Autodesk Fusion 360 part; units mm, degrees
(part 3 of 5)
  spline S134 degree 5 poles (-1.9006, 45.6475) (-1.9013, 45.6491) (-1.9092, 45.6653) (-1.9241, 45.6961) (-1.9463, 45.7414) (-1.9758, 45.8013) (-2.0121, 45.8741) (-2.0487, 45.9468) (-2.0857, 46.0195) (-2.123, 46.092) (-2.1607, 46.1645) (-2.1987, 46.2369) (-2.2371, 46.3092) (-2.2758, 46.3814) (-2.3148, 46.4536) (-2.3542, 46.5256) (-2.3938, 46.5976) (-2.4339, 46.6694) (-2.4742, 46.7412) (-2.5149, 46.8129) (-2.5559, 46.8845) (-2.5972, 46.956) (-2.6305, 47.0132) (-2.6556, 47.056) (-2.6724, 47.0845) (-2.6809, 47.0988) knots 0.712736 0.712736 0.712736 0.712736 0.712736 0.712736 0.714286 0.728571 0.742857 0.757143 0.771429 0.785714 0.8 0.814286 0.828571 0.842857 0.857143 0.871429 0.885714 0.9 0.914286 0.928571 0.942857 0.957143 0.971429 0.985714 1 1 1 1 1 1
  arc A101 (-2.6809, 47.0988) -> (-3.2433, 47.0634) centre (0, 0) ccw
  spline S135 degree 5 poles (-44.9524, 14.3096) (-44.9406, 14.2979) (-44.9172, 14.2745) (-44.882, 14.2396) (-44.8349, 14.1931) (-44.7759, 14.1353) (-44.7168, 14.0778) (-44.6574, 14.0206) (-44.5979, 13.9636) (-44.5383, 13.907) (-44.4785, 13.8506) (-44.4185, 13.7946) (-44.3583, 13.7389) (-44.298, 13.6834) (-44.2375, 13.6283) (-44.1768, 13.5735) (-44.116, 13.5189) (-44.055, 13.4647) (-43.9938, 13.4109) (-43.9325, 13.3573) (-43.871, 13.3041) (-43.8203, 13.2606) (-43.7819, 13.2278) (-43.7558, 13.2057) (-43.7421, 13.1941) (-43.7407, 13.1929) knots -1 -1 -1 -1 -1 -1 -0.985714 -0.971429 -0.957143 -0.942857 -0.928571 -0.914286 -0.9 -0.885714 -0.871429 -0.857143 -0.842857 -0.828571 -0.814286 -0.8 -0.785714 -0.771429 -0.757143 -0.742857 -0.728571 -0.714286 -0.712736 -0.712736 -0.712736 -0.712736 -0.712736 -0.712736
  spline S136 degree 5 poles (-22.8544, -39.5598) (-22.8546, -39.5616) (-22.8567, -39.5795) (-22.8606, -39.6135) (-22.8662, -39.6636) (-22.8733, -39.73) (-22.8817, -39.8109) (-22.8898, -39.892) (-22.8975, -39.9731) (-22.9048, -40.0544) (-22.9118, -40.1357) (-22.9185, -40.2172) (-22.9249, -40.2988) (-22.9309, -40.3805) (-22.9366, -40.4624) (-22.942, -40.5443) (-22.947, -40.6263) (-22.9517, -40.7084) (-22.9561, -40.7907) (-22.9602, -40.873) (-22.964, -40.9554) (-22.9674, -41.0379) (-22.9699, -41.104) (-22.9716, -41.1536) (-22.9727, -41.1867) (-22.9733, -41.2033) knots 0.712736 0.712736 0.712736 0.712736 0.712736 0.712736 0.714286 0.728571 0.742857 0.757143 0.771429 0.785714 0.8 0.814286 0.828571 0.842857 0.857143 0.871429 0.885714 0.9 0.914286 0.928571 0.942857 0.957143 0.971429 0.985714 1 1 1 1 1 1
  spline S137 degree 5 poles (22.4794, 41.4748) (22.4657, 41.4655) (22.4383, 41.4468) (22.3974, 41.4188) (22.3429, 41.3812) (22.2751, 41.3341) (22.2075, 41.2868) (22.1402, 41.2392) (22.0731, 41.1915) (22.0063, 41.1435) (21.9397, 41.0953) (21.8734, 41.0468) (21.8074, 40.9982) (21.7417, 40.9493) (21.6762, 40.9002) (21.6109, 40.8509) (21.546, 40.8014) (21.4813, 40.7516) (21.4169, 40.7016) (21.3528, 40.6514) (21.289, 40.601) (21.2368, 40.5594) (21.1974, 40.5278) (21.1708, 40.5063) (21.1568, 40.495) (21.1555, 40.4939) knots -1 -1 -1 -1 -1 -1 -0.985714 -0.971429 -0.957143 -0.942857 -0.928571 -0.914286 -0.9 -0.885714 -0.871429 -0.857143 -0.842857 -0.828571 -0.814286 -0.8 -0.785714 -0.771429 -0.757143 -0.742857 -0.728571 -0.714286 -0.712736 -0.712736 -0.712736 -0.712736 -0.712736 -0.712736
  spline S138 degree 5 poles (-17.628, 43.7577) (-17.6295, 43.7412) (-17.6326, 43.7082) (-17.6371, 43.6588) (-17.6429, 43.5929) (-17.6498, 43.5106) (-17.6564, 43.4284) (-17.6627, 43.3462) (-17.6686, 43.264) (-17.6743, 43.182) (-17.6795, 43.1) (-17.6845, 43.018) (-17.6891, 42.9361) (-17.6933, 42.8543) (-17.6973, 42.7726) (-17.7008, 42.6909) (-17.7041, 42.6093) (-17.707, 42.5277) (-17.7095, 42.4462) (-17.7117, 42.3648) (-17.7135, 42.2835) (-17.7147, 42.2168) (-17.7154, 42.1663) (-17.7158, 42.1321) (-17.716, 42.1141) (-17.7161, 42.1123) knots -1 -1 -1 -1 -1 -1 -0.985714 -0.971429 -0.957143 -0.942857 -0.928571 -0.914286 -0.9 -0.885714 -0.871429 -0.857143 -0.842857 -0.828571 -0.814286 -0.8 -0.785714 -0.771429 -0.757143 -0.742857 -0.728571 -0.714286 -0.712736 -0.712736 -0.712736 -0.712736 -0.712736 -0.712736
  spline S139 degree 3 poles (-42.1123, 17.7161) (-42.0459, 17.7168) (-41.9803, 17.7305) (-41.858, 17.7822) (-41.8024, 17.8198) (-41.7089, 17.9141) (-41.6718, 17.97) (-41.6211, 18.0927) (-41.608, 18.1585) (-41.6077, 18.2913) (-41.6206, 18.3571) (-41.6685, 18.4748) (-41.7013, 18.5264) (-41.7423, 18.5711) knots 0 0 0 0 0.019923 0.019923 0.039846 0.039846 0.059769 0.059769 0.079691 0.079691 0.099614 0.099614 0.117812 0.117812 0.117812 0.117812
  arc A102 (-8.5628, 46.3914) -> (-9.1163, 46.2858) centre (0, 0) ccw
  spline S140 degree 3 poles (27.6324, 36.3835) (27.6166, 36.319) (27.6135, 36.252) (27.6332, 36.1207) (27.6558, 36.0575) (27.7239, 35.9435) (27.7688, 35.8937) (27.8751, 35.8141) (27.9355, 35.785) (28.0641, 35.7517) (28.131, 35.7477) (28.2569, 35.7649) (28.3151, 35.7838) (28.3685, 35.8125) knots 0 0 0 0 0.019923 0.019923 0.039846 0.039846 0.059769 0.059769 0.079691 0.079691 0.099614 0.099614 0.117812 0.117812 0.117812 0.117812
  spline S141 degree 5 poles (-45.5258, 3.8356) (-45.5274, 3.835) (-45.5445, 3.8292) (-45.5769, 3.8183) (-45.6247, 3.802) (-45.6878, 3.7802) (-45.7646, 3.7533) (-45.8413, 3.7261) (-45.918, 3.6985) (-45.9947, 3.6706) (-46.0713, 3.6423) (-46.1479, 3.6137) (-46.2244, 3.5847) (-46.3009, 3.5553) (-46.3774, 3.5256) (-46.4538, 3.4956) (-46.5301, 3.4653) (-46.6065, 3.4346) (-46.6827, 3.4035) (-46.759, 3.3722) (-46.8351, 3.3405) (-46.9113, 3.3084) (-46.9721, 3.2825) (-47.0178, 3.263) (-47.0482, 3.2499) (-47.0634, 3.2433) knots 0.712736 0.712736 0.712736 0.712736 0.712736 0.712736 0.714286 0.728571 0.742857 0.757143 0.771429 0.785714 0.8 0.814286 0.828571 0.842857 0.857143 0.871429 0.885714 0.9 0.914286 0.928571 0.942857 0.957143 0.971429 0.985714 1 1 1 1 1 1
  spline S142 degree 5 poles (-42.1123, 17.7161) (-42.1141, 17.716) (-42.1321, 17.7158) (-42.1663, 17.7154) (-42.2168, 17.7147) (-42.2835, 17.7135) (-42.3648, 17.7117) (-42.4462, 17.7095) (-42.5277, 17.707) (-42.6093, 17.7041) (-42.6909, 17.7008) (-42.7726, 17.6973) (-42.8543, 17.6933) (-42.9361, 17.6891) (-43.018, 17.6845) (-43.1, 17.6795) (-43.182, 17.6743) (-43.264, 17.6686) (-43.3462, 17.6627) (-43.4284, 17.6564) (-43.5106, 17.6498) (-43.5929, 17.6429) (-43.6588, 17.6371) (-43.7082, 17.6326) (-43.7412, 17.6295) (-43.7577, 17.628) knots 0.712736 0.712736 0.712736 0.712736 0.712736 0.712736 0.714286 0.728571 0.742857 0.757143 0.771429 0.785714 0.8 0.814286 0.828571 0.842857 0.857143 0.871429 0.885714 0.9 0.914286 0.928571 0.942857 0.957143 0.971429 0.985714 1 1 1 1 1 1
  spline S143 degree 3 poles (22.8544, 39.5598) (22.8468, 39.4939) (22.8522, 39.427) (22.8882, 39.2992) (22.9185, 39.2394) (23.0004, 39.1348) (23.0511, 39.091) (23.1666, 39.0253) (23.2302, 39.0041) (23.3619, 38.9871) (23.4288, 38.9916) (23.5515, 39.0245) (23.6069, 39.0505) (23.6563, 39.0856) knots 0 0 0 0 0.019923 0.019923 0.039846 0.039846 0.059769 0.059769 0.079691 0.079691 0.099614 0.099614 0.117812 0.117812 0.117812 0.117812
  spline S144 degree 5 poles (22.8544, 39.5598) (22.8546, 39.5616) (22.8567, 39.5795) (22.8606, 39.6135) (22.8662, 39.6636) (22.8733, 39.73) (22.8817, 39.8109) (22.8898, 39.892) (22.8975, 39.9731) (22.9048, 40.0544) (22.9118, 40.1357) (22.9185, 40.2172) (22.9249, 40.2988) (22.9309, 40.3805) (22.9366, 40.4624) (22.942, 40.5443) (22.947, 40.6263) (22.9517, 40.7084) (22.9561, 40.7907) (22.9602, 40.873) (22.964, 40.9554) (22.9674, 41.0379) (22.9699, 41.104) (22.9716, 41.1536) (22.9727, 41.1867) (22.9733, 41.2033) knots 0.712736 0.712736 0.712736 0.712736 0.712736 0.712736 0.714286 0.728571 0.742857 0.757143 0.771429 0.785714 0.8 0.814286 0.828571 0.842857 0.857143 0.871429 0.885714 0.9 0.914286 0.928571 0.942857 0.957143 0.971429 0.985714 1 1 1 1 1 1
  spline S145 degree 3 poles (-22.8544, -39.5598) (-22.8468, -39.4939) (-22.8522, -39.427) (-22.8882, -39.2992) (-22.9185, -39.2394) (-23.0004, -39.1348) (-23.0511, -39.091) (-23.1666, -39.0253) (-23.2302, -39.0041) (-23.3619, -38.9871) (-23.4288, -38.9916) (-23.5515, -39.0245) (-23.6069, -39.0505) (-23.6563, -39.0856) knots 0 0 0 0 0.019923 0.019923 0.039846 0.039846 0.059769 0.059769 0.079691 0.079691 0.099614 0.099614 0.117812 0.117812 0.117812 0.117812
  spline S146 degree 5 poles (-44.0007, 12.2983) (-44.0024, 12.2981) (-44.0202, 12.2956) (-44.0541, 12.2909) (-44.1041, 12.2838) (-44.1702, 12.2743) (-44.2506, 12.2623) (-44.3311, 12.2499) (-44.4116, 12.2372) (-44.4922, 12.2241) (-44.5727, 12.2107) (-44.6533, 12.1969) (-44.734, 12.1828) (-44.8146, 12.1683) (-44.8953, 12.1534) (-44.9759, 12.1383) (-45.0566, 12.1228) (-45.1374, 12.1069) (-45.2181, 12.0907) (-45.2989, 12.0742) (-45.3796, 12.0573) (-45.4604, 12.0401) (-45.525, 12.0261) (-45.5735, 12.0154) (-45.6059, 12.0083) (-45.622, 12.0047) knots 0.712736 0.712736 0.712736 0.712736 0.712736 0.712736 0.714286 0.728571 0.742857 0.757143 0.771429 0.785714 0.8 0.814286 0.828571 0.842857 0.857143 0.871429 0.885714 0.9 0.914286 0.928571 0.942857 0.957143 0.971429 0.985714 1 1 1 1 1 1
  spline S147 degree 5 poles (-6.192, 46.7669) (-6.1976, 46.7513) (-6.2088, 46.7201) (-6.2255, 46.6733) (-6.2475, 46.611) (-6.2747, 46.533) (-6.3015, 46.455) (-6.328, 46.3769) (-6.3542, 46.2988) (-6.3801, 46.2207) (-6.4056, 46.1426) (-6.4307, 46.0645) (-6.4556, 45.9863) (-6.48, 45.9081) (-6.5042, 45.8299) (-6.5279, 45.7517) (-6.5514, 45.6734) (-6.5744, 45.5952) (-6.5972, 45.5169) (-6.6195, 45.4386) (-6.6415, 45.3603) (-6.6593, 45.2959) (-6.6725, 45.2472) (-6.6815, 45.2142) (-6.6861, 45.1968) (-6.6866, 45.1951) knots -1 -1 -1 -1 -1 -1 -0.985714 -0.971429 -0.957143 -0.942857 -0.928571 -0.914286 -0.9 -0.885714 -0.871429 -0.857143 -0.842857 -0.828571 -0.814286 -0.8 -0.785714 -0.771429 -0.757143 -0.742857 -0.728571 -0.714286 -0.712736 -0.712736 -0.712736 -0.712736 -0.712736 -0.712736
  arc A103 (-34.5814, -32.0875) -> (-34.1956, -32.4983) centre (0, 0) ccw
  arc A104 (-27.9562, -37.9991) -> (-27.5003, -38.3303) centre (0, 0) ccw
  spline S148 degree 5 poles (27.5003, 38.3303) (27.4856, 38.3228) (27.4561, 38.3077) (27.4119, 38.285) (27.3532, 38.2546) (27.28, 38.2164) (27.207, 38.1779) (27.1342, 38.1392) (27.0617, 38.1002) (26.9894, 38.0609) (26.9173, 38.0214) (26.8455, 37.9817) (26.7739, 37.9417) (26.7025, 37.9015) (26.6314, 37.861) (26.5605, 37.8202) (26.4899, 37.7792) (26.4195, 37.738) (26.3493, 37.6964) (26.2794, 37.6547) (26.2098, 37.6126) (26.1528, 37.5779) (26.1098, 37.5514) (26.0807, 37.5335) (26.0654, 37.524) (26.0639, 37.5231) knots -1 -1 -1 -1 -1 -1 -0.985714 -0.971429 -0.957143 -0.942857 -0.928571 -0.914286 -0.9 -0.885714 -0.871429 -0.857143 -0.842857 -0.828571 -0.814286 -0.8 -0.785714 -0.771429 -0.757143 -0.742857 -0.728571 -0.714286 -0.712736 -0.712736 -0.712736 -0.712736 -0.712736 -0.712736
  spline S149 degree 5 poles (-3.2433, 47.0634) (-3.2499, 47.0482) (-3.263, 47.0178) (-3.2825, 46.9721) (-3.3084, 46.9113) (-3.3405, 46.8351) (-3.3722, 46.759) (-3.4035, 46.6827) (-3.4346, 46.6065) (-3.4653, 46.5301) (-3.4956, 46.4538) (-3.5256, 46.3774) (-3.5553, 46.3009) (-3.5847, 46.2244) (-3.6137, 46.1479) (-3.6423, 46.0713) (-3.6706, 45.9947) (-3.6985, 45.918) (-3.7261, 45.8413) (-3.7533, 45.7646) (-3.7802, 45.6878) (-3.802, 45.6247) (-3.8183, 45.5769) (-3.8292, 45.5445) (-3.835, 45.5274) (-3.8356, 45.5258) knots -1 -1 -1 -1 -1 -1 -0.985714 -0.971429 -0.957143 -0.942857 -0.928571 -0.914286 -0.9 -0.885714 -0.871429 -0.857143 -0.842857 -0.828571 -0.814286 -0.8 -0.785714 -0.771429 -0.757143 -0.742857 -0.728571 -0.714286 -0.712736 -0.712736 -0.712736 -0.712736 -0.712736 -0.712736
  arc A105 (45.7622, 11.4588) -> (45.622, 12.0047) centre (0, 0) ccw
  spline S150 degree 3 poles (43.7407, 13.1929) (43.69, 13.1501) (43.6482, 13.0977) (43.5869, 12.9798) (43.5681, 12.9155) (43.5562, 12.7832) (43.5632, 12.7165) (43.6024, 12.5896) (43.6342, 12.5306) (43.7186, 12.4281) (43.7704, 12.3855) (43.8824, 12.3255) (43.9406, 12.3066) (44.0007, 12.2983) knots 0 0 0 0 0.019923 0.019923 0.039846 0.039846 0.059769 0.059769 0.079691 0.079691 0.099614 0.099614 0.117812 0.117812 0.117812 0.117812
  spline S151 degree 5 poles (44.7782, 14.8456) (44.7619, 14.8482) (44.7291, 14.8533) (44.6801, 14.8609) (44.6147, 14.8709) (44.533, 14.8829) (44.4513, 14.8947) (44.3697, 14.9061) (44.2881, 14.9172) (44.2065, 14.928) (44.125, 14.9384) (44.0436, 14.9485) (43.9621, 14.9582) (43.8807, 14.9676) (43.7994, 14.9766) (43.7181, 14.9853) (43.6368, 14.9937) (43.5556, 15.0017) (43.4745, 15.0093) (43.3934, 15.0166) (43.3123, 15.0235) (43.2458, 15.0289) (43.1954, 15.0328) (43.1613, 15.0354) (43.1434, 15.0367) (43.1416, 15.0368) knots -1 -1 -1 -1 -1 -1 -0.985714 -0.971429 -0.957143 -0.942857 -0.928571 -0.914286 -0.9 -0.885714 -0.871429 -0.857143 -0.842857 -0.828571 -0.814286 -0.8 -0.785714 -0.771429 -0.757143 -0.742857 -0.728571 -0.714286 -0.712736 -0.712736 -0.712736 -0.712736 -0.712736 -0.712736
  arc A106 (42.8044, 19.8308) -> (42.5645, 20.3407) centre (0, 0) ccw
  line L56 (29.0727, 9.9241) -> (36.6833, 12.3969)
  spline S152 degree 5 poles (44.4828, 10.4204) (44.4842, 10.4215) (44.4987, 10.4322) (44.5261, 10.4526) (44.5665, 10.4829) (44.6198, 10.5231) (44.6845, 10.5724) (44.7491, 10.622) (44.8135, 10.6719) (44.8778, 10.7222) (44.9419, 10.7728) (45.0059, 10.8237) (45.0698, 10.8749) (45.1334, 10.9265) (45.197, 10.9783) (45.2604, 11.0305) (45.3236, 11.083) (45.3867, 11.1357) (45.4497, 11.1888) (45.5125, 11.2422) (45.5751, 11.2959) (45.6376, 11.3499) (45.6875, 11.3933) (45.7249, 11.426) (45.7497, 11.4479) (45.7622, 11.4588) knots 0.712736 0.712736 0.712736 0.712736 0.712736 0.712736 0.714286 0.728571 0.742857 0.757143 0.771429 0.785714 0.8 0.814286 0.828571 0.842857 0.857143 0.871429 0.885714 0.9 0.914286 0.928571 0.942857 0.957143 0.971429 0.985714 1 1 1 1 1 1
  line L57 (23.3964, 19.6289) -> (29.5622, 24.7297)
  line L58 (25.6911, 16.6409) -> (32.4476, 20.9287)
  spline S153 degree 5 poles (40.4939, 21.1555) (40.495, 21.1568) (40.5063, 21.1708) (40.5278, 21.1974) (40.5594, 21.2368) (40.601, 21.289) (40.6514, 21.3528) (40.7016, 21.4169) (40.7516, 21.4813) (40.8014, 21.546) (40.8509, 21.6109) (40.9002, 21.6762) (40.9493, 21.7417) (40.9982, 21.8074) (41.0468, 21.8734) (41.0953, 21.9397) (41.1435, 22.0063) (41.1915, 22.0731) (41.2392, 22.1402) (41.2868, 22.2075) (41.3341, 22.2751) (41.3812, 22.3429) (41.4188, 22.3974) (41.4468, 22.4383) (41.4655, 22.4657) (41.4748, 22.4794) knots 0.712736 0.712736 0.712736 0.712736 0.712736 0.712736 0.714286 0.728571 0.742857 0.757143 0.771429 0.785714 0.8 0.814286 0.828571 0.842857 0.857143 0.871429 0.885714 0.9 0.914286 0.928571 0.942857 0.957143 0.971429 0.985714 1 1 1 1 1 1
  arc A107 (-11.213, -27.5925) -> (-9.5008, -28.2786) centre (0.7975, -0.1016) ccw
  spline S154 degree 3 poles (39.0856, 23.6563) (39.0471, 23.6022) (39.0196, 23.541) (38.9896, 23.4117) (38.9874, 23.3447) (39.0087, 23.2136) (39.0321, 23.1507) (39.1016, 23.0376) (39.1471, 22.9883) (39.2544, 22.91) (39.3152, 22.8817) (39.4386, 22.8514) (39.4996, 22.8475) (39.5598, 22.8544) knots 0 0 0 0 0.019923 0.019923 0.039846 0.039846 0.059769 0.059769 0.079691 0.079691 0.099614 0.099614 0.117812 0.117812 0.117812 0.117812
  arc A108 (43.9652, 17.104) -> (43.7577, 17.628) centre (0, 0) ccw
  spline S155 degree 3 poles (42.826, 15.9134) (42.7781, 15.8674) (42.7397, 15.8125) (42.6859, 15.6911) (42.6712, 15.6257) (42.6676, 15.4929) (42.6788, 15.4268) (42.7258, 15.3026) (42.7613, 15.2457) (42.852, 15.1487) (42.9064, 15.1095) (43.0219, 15.0565) (43.0811, 15.0413) (43.1416, 15.0368) knots 0 0 0 0 0.019923 0.019923 0.039846 0.039846 0.059769 0.059769 0.079691 0.079691 0.099614 0.099614 0.117812 0.117812 0.117812 0.117812
  arc A109 (33.573, 19.1277) -> (32.4476, 20.9287) centre (0.7975, -0.1016) ccw
  spline S156 degree 5 poles (45.6768, -0.9694) (45.6784, -0.9687) (45.695, -0.9619) (45.7267, -0.9489) (45.7734, -0.9297) (45.835, -0.904) (45.9099, -0.8723) (45.9848, -0.8404) (46.0596, -0.808) (46.1344, -0.7753) (46.2091, -0.7423) (46.2837, -0.7089) (46.3583, -0.6751) (46.4328, -0.641) (46.5072, -0.6066) (46.5816, -0.5719) (46.6559, -0.5368) (46.7302, -0.5013) (46.8043, -0.4656) (46.8784, -0.4295) (46.9525, -0.3931) (47.0264, -0.3563) (47.0856, -0.3267) (47.1299, -0.3043) (47.1594, -0.2893) (47.1742, -0.2818) knots 0.712736 0.712736 0.712736 0.712736 0.712736 0.712736 0.714286 0.728571 0.742857 0.757143 0.771429 0.785714 0.8 0.814286 0.828571 0.842857 0.857143 0.871429 0.885714 0.9 0.914286 0.928571 0.942857 0.957143 0.971429 0.985714 1 1 1 1 1 1
  line L59 (27.5932, 13.3889) -> (34.8338, 16.7961)
  line L60 (28.3716, 11.7167) -> (35.7247, 14.8682)
  arc A110 (-47.1742, 0.2818) -> (-47.1742, -0.2818) centre (0, 0) ccw
  arc A111 (37.3255, 10.3726) -> (36.6833, 12.3969) centre (0.7975, -0.1016) ccw
  spline S157 degree 5 poles (42.826, 15.9134) (42.8273, 15.9146) (42.8403, 15.9271) (42.8649, 15.9508) (42.9012, 15.9859) (42.9491, 16.0325) (43.0071, 16.0895) (43.065, 16.1468) (43.1226, 16.2044) (43.1801, 16.2623) (43.2374, 16.3206) (43.2945, 16.3791) (43.3514, 16.4379) (43.4081, 16.497) (43.4646, 16.5564) (43.521, 16.6161) (43.5772, 16.6761) (43.6332, 16.7364) (43.689, 16.7969) (43.7446, 16.8578) (43.8, 16.9189) (43.8553, 16.9803) (43.8993, 17.0296) (43.9323, 17.0668) (43.9542, 17.0916) (43.9652, 17.104) knots 0.712736 0.712736 0.712736 0.712736 0.712736 0.712736 0.714286 0.728571 0.742857 0.757143 0.771429 0.785714 0.8 0.814286 0.828571 0.842857 0.857143 0.871429 0.885714 0.9 0.914286 0.928571 0.942857 0.957143 0.971429 0.985714 1 1 1 1 1 1
  line L61 (0.7975, -0.1016) -> (38, -0.1016) construction
  line L62 (24.5662, 18.2028) -> (30.9045, 23.0839)
  arc A112 (44.9524, 14.3096) -> (44.7782, 14.8456) centre (0, 0) ccw
  spline S158 degree 5 poles (41.7423, 18.5711) (41.7435, 18.5724) (41.7557, 18.5856) (41.7788, 18.6109) (41.8128, 18.6481) (41.8576, 18.6976) (41.912, 18.7582) (41.9661, 18.819) (42.02, 18.8801) (42.0738, 18.9415) (42.1273, 19.0032) (42.1806, 19.0652) (42.2337, 19.1275) (42.2866, 19.1901) (42.3393, 19.2529) (42.3918, 19.3161) (42.4441, 19.3794) (42.4962, 19.4431) (42.5481, 19.5071) (42.5997, 19.5713) (42.6512, 19.6357) (42.7025, 19.7005) (42.7434, 19.7525) (42.7739, 19.7916) (42.7943, 19.8177) (42.8044, 19.8308) knots 0.712736 0.712736 0.712736 0.712736 0.712736 0.712736 0.714286 0.728571 0.742857 0.757143 0.771429 0.785714 0.8 0.814286 0.828571 0.842857 0.857143 0.871429 0.885714 0.9 0.914286 0.928571 0.942857 0.957143 0.971429 0.985714 1 1 1 1 1 1
  line L63 (26.6729, 15.0794) -> (33.573, 19.1277)
  spline S159 degree 5 poles (45.4381, 4.7631) (45.4396, 4.7639) (45.4553, 4.7728) (45.4851, 4.7896) (45.5289, 4.8146) (45.5869, 4.8478) (45.6572, 4.8886) (45.7275, 4.9297) (45.7977, 4.9712) (45.8678, 5.013) (45.9377, 5.0551) (46.0076, 5.0976) (46.0774, 5.1404) (46.147, 5.1836) (46.2165, 5.2271) (46.286, 5.2709) (46.3553, 5.315) (46.4245, 5.3595) (46.4936, 5.4042) (46.5626, 5.4493) (46.6315, 5.4947) (46.7003, 5.5405) (46.7552, 5.5773) (46.7964, 5.6051) (46.8238, 5.6236) (46.8375, 5.6329) knots 0.712736 0.712736 0.712736 0.712736 0.712736 0.712736 0.714286 0.728571 0.742857 0.757143 0.771429 0.785714 0.8 0.814286 0.828571 0.842857 0.857143 0.871429 0.885714 0.9 0.914286 0.928571 0.942857 0.957143 0.971429 0.985714 1 1 1 1 1 1
  arc A113 (47.1742, -0.2818) -> (47.1742, 0.2818) centre (0, 0) ccw
  arc A114 (38.3502, 5.7119) -> (37.9668, 7.8007) centre (0.7975, -0.1016) ccw
  spline S160 degree 5 poles (47.0634, 3.2433) (47.0482, 3.2499) (47.0178, 3.263) (46.9721, 3.2825) (46.9113, 3.3084) (46.8351, 3.3405) (46.759, 3.3722) (46.6827, 3.4035) (46.6065, 3.4346) (46.5301, 3.4653) (46.4538, 3.4956) (46.3774, 3.5256) (46.3009, 3.5553) (46.2244, 3.5847) (46.1479, 3.6137) (46.0713, 3.6423) (45.9947, 3.6706) (45.918, 3.6985) (45.8413, 3.7261) (45.7646, 3.7533) (45.6878, 3.7802) (45.6247, 3.802) (45.5769, 3.8183) (45.5445, 3.8292) (45.5274, 3.835) (45.5258, 3.8356) knots -1 -1 -1 -1 -1 -1 -0.985714 -0.971429 -0.957143 -0.942857 -0.928571 -0.914286 -0.9 -0.885714 -0.871429 -0.857143 -0.842857 -0.828571 -0.814286 -0.8 -0.785714 -0.771429 -0.757143 -0.742857 -0.728571 -0.714286 -0.712736 -0.712736 -0.712736 -0.712736 -0.712736 -0.712736
  arc A115 (30.4444, 4.488) -> (30.1063, 6.3012) centre (0.7975, -0.1016) ccw
  spline S161 degree 3 poles (45.4381, 4.7631) (45.3802, 4.7304) (45.3293, 4.6868) (45.2471, 4.5825) (45.2165, 4.5229) (45.18, 4.3952) (45.1744, 4.3283) (45.1891, 4.1963) (45.2093, 4.1324) (45.273, 4.0159) (45.316, 3.9644) (45.4147, 3.8844) (45.4683, 3.8549) (45.5258, 3.8356) knots 0 0 0 0 0.019923 0.019923 0.039846 0.039846 0.059769 0.059769 0.079691 0.079691 0.099614 0.099614 0.117812 0.117812 0.117812 0.117812
  arc A116 (47.0988, 2.6809) -> (47.0634, 3.2433) centre (0, 0) ccw
  spline S162 degree 5 poles (45.0493, 7.6067) (45.0508, 7.6077) (45.0659, 7.6175) (45.0946, 7.6362) (45.1368, 7.6639) (45.1925, 7.7007) (45.2602, 7.7458) (45.3278, 7.7912) (45.3952, 7.837) (45.4625, 7.8831) (45.5297, 7.9296) (45.5967, 7.9764) (45.6637, 8.0235) (45.7305, 8.0709) (45.7971, 8.1187) (45.8637, 8.1668) (45.9301, 8.2152) (45.9964, 8.2639) (46.0625, 8.3129) (46.1286, 8.3623) (46.1945, 8.4119) (46.2602, 8.4619) (46.3128, 8.5021) (46.3521, 8.5324) (46.3783, 8.5526) (46.3914, 8.5628) knots 0.712736 0.712736 0.712736 0.712736 0.712736 0.712736 0.714286 0.728571 0.742857 0.757143 0.771429 0.785714 0.8 0.814286 0.828571 0.842857 0.857143 0.871429 0.885714 0.9 0.914286 0.928571 0.942857 0.957143 0.971429 0.985714 1 1 1 1 1 1
  spline S163 degree 5 poles (46.2858, 9.1163) (46.2699, 9.121) (46.2381, 9.1301) (46.1903, 9.1438) (46.1267, 9.1619) (46.0472, 9.1841) (45.9676, 9.206) (45.8881, 9.2276) (45.8085, 9.2488) (45.7289, 9.2697) (45.6494, 9.2903) (45.5698, 9.3105) (45.4902, 9.3303) (45.4106, 9.3498) (45.3311, 9.369) (45.2515, 9.3878) (45.1719, 9.4063) (45.0924, 9.4244) (45.0128, 9.4422) (44.9333, 9.4596) (44.8537, 9.4766) (44.7884, 9.4903) (44.7389, 9.5005) (44.7054, 9.5073) (44.6878, 9.5109) (44.686, 9.5112) knots -1 -1 -1 -1 -1 -1 -0.985714 -0.971429 -0.957143 -0.942857 -0.928571 -0.914286 -0.9 -0.885714 -0.871429 -0.857143 -0.842857 -0.828571 -0.814286 -0.8 -0.785714 -0.771429 -0.757143 -0.742857 -0.728571 -0.714286 -0.712736 -0.712736 -0.712736 -0.712736 -0.712736 -0.712736
  spline S164 degree 5 poles (47.1742, 0.2818) (47.1594, 0.2893) (47.1299, 0.3043) (47.0856, 0.3267) (47.0264, 0.3563) (46.9525, 0.3931) (46.8784, 0.4295) (46.8043, 0.4656) (46.7302, 0.5013) (46.6559, 0.5368) (46.5816, 0.5719) (46.5072, 0.6066) (46.4328, 0.641) (46.3583, 0.6751) (46.2837, 0.7089) (46.2091, 0.7423) (46.1344, 0.7753) (46.0596, 0.808) (45.9848, 0.8404) (45.9099, 0.8723) (45.835, 0.904) (45.7734, 0.9297) (45.7267, 0.9489) (45.695, 0.9619) (45.6784, 0.9687) (45.6768, 0.9694) knots -1 -1 -1 -1 -1 -1 -0.985714 -0.971429 -0.957143 -0.942857 -0.928571 -0.914286 -0.9 -0.885714 -0.871429 -0.857143 -0.842857 -0.828571 -0.814286 -0.8 -0.785714 -0.771429 -0.757143 -0.742857 -0.728571 -0.714286 -0.712736 -0.712736 -0.712736 -0.712736 -0.712736 -0.712736
  spline S165 degree 3 poles (44.4828, 10.4204) (44.4295, 10.3808) (44.3845, 10.3311) (44.3159, 10.2174) (44.2931, 10.1543) (44.2729, 10.0231) (44.2757, 9.9561) (44.3069, 9.827) (44.3349, 9.7661) (44.4127, 9.6584) (44.4618, 9.6127) (44.5698, 9.5457) (44.6266, 9.5232) (44.686, 9.5112) knots 0 0 0 0 0.019923 0.019923 0.039846 0.039846 0.059769 0.059769 0.079691 0.079691 0.099614 0.099614 0.117812 0.117812 0.117812 0.117812
  line L64 (30.6777, 2.5774) -> (38.6641, 3.0798)
  line L65 (30.1063, 6.3012) -> (37.9668, 7.8007)
  line L66 (30.4444, 4.488) -> (38.3502, 5.7119)
  line L67 (30.7858, 0.736) -> (38.7827, 0.9594)
  arc A117 (38.7827, 0.9594) -> (38.6641, 3.0798) centre (0.7975, -0.1016) ccw
  arc A118 (46.3914, 8.5628) -> (46.2858, 9.1163) centre (0, 0) ccw
  arc A119 (29.6354, 8.1675) -> (29.0727, 9.9241) centre (0.7975, -0.1016) ccw
  spline S166 degree 3 poles (45.0493, 7.6067) (44.9937, 7.5705) (44.9456, 7.5238) (44.87, 7.4146) (44.8433, 7.3531) (44.8149, 7.2234) (44.8135, 7.1563) (44.8365, 7.0255) (44.8606, 6.963) (44.9315, 6.8507) (44.9776, 6.802) (45.0812, 6.7283) (45.1365, 6.7023) (45.1951, 6.6866) knots 0 0 0 0 0.019923 0.019923 0.039846 0.039846 0.059769 0.059769 0.079691 0.079691 0.099614 0.099614 0.117812 0.117812 0.117812 0.117812
  spline S167 degree 3 poles (45.6475, 1.9006) (45.5877, 1.8717) (45.5342, 1.8313) (45.4455, 1.7324) (45.4113, 1.6748) (45.3668, 1.5496) (45.3571, 1.4833) (45.3634, 1.3506) (45.3796, 1.2855) (45.4359, 1.1652) (45.4755, 1.1112) (45.569, 1.0251) (45.6206, 0.9923) (45.6768, 0.9694) knots 0 0 0 0 0.019923 0.019923 0.039846 0.039846 0.059769 0.059769 0.079691 0.079691 0.099614 0.099614 0.117812 0.117812 0.117812 0.117812
  spline S168 degree 5 poles (42.5645, 20.3407) (42.5479, 20.3413) (42.5148, 20.3422) (42.4652, 20.3436) (42.3991, 20.3453) (42.3165, 20.347) (42.234, 20.3485) (42.1516, 20.3496) (42.0693, 20.3504) (41.987, 20.3508) (41.9048, 20.3509) (41.8227, 20.3507) (41.7407, 20.3502) (41.6588, 20.3493) (41.5769, 20.3481) (41.4952, 20.3465) (41.4135, 20.3446) (41.332, 20.3423) (41.2505, 20.3398) (41.1691, 20.3368) (41.0878, 20.3335) (41.0211, 20.3305) (40.9707, 20.3281) (40.9365, 20.3264) (40.9186, 20.3254) (40.9168, 20.3254) knots -1 -1 -1 -1 -1 -1 -0.985714 -0.971429 -0.957143 -0.942857 -0.928571 -0.914286 -0.9 -0.885714 -0.871429 -0.857143 -0.842857 -0.828571 -0.814286 -0.8 -0.785714 -0.771429 -0.757143 -0.742857 -0.728571 -0.714286 -0.712736 -0.712736 -0.712736 -0.712736 -0.712736 -0.712736
  spline S169 degree 5 poles (45.622, 12.0047) (45.6059, 12.0083) (45.5735, 12.0154) (45.525, 12.0261) (45.4604, 12.0401) (45.3796, 12.0573) (45.2989, 12.0742) (45.2181, 12.0907) (45.1374, 12.1069) (45.0566, 12.1228) (44.9759, 12.1383) (44.8953, 12.1534) (44.8146, 12.1683) (44.734, 12.1828) (44.6533, 12.1969) (44.5727, 12.2107) (44.4922, 12.2241) (44.4116, 12.2372) (44.3311, 12.2499) (44.2506, 12.2623) (44.1702, 12.2743) (44.1041, 12.2838) (44.0541, 12.2909) (44.0202, 12.2956) (44.0024, 12.2981) (44.0007, 12.2983) knots -1 -1 -1 -1 -1 -1 -0.985714 -0.971429 -0.957143 -0.942857 -0.928571 -0.914286 -0.9 -0.885714 -0.871429 -0.857143 -0.842857 -0.828571 -0.814286 -0.8 -0.785714 -0.771429 -0.757143 -0.742857 -0.728571 -0.714286 -0.712736 -0.712736 -0.712736 -0.712736 -0.712736 -0.712736
  arc A120 (41.4748, 22.4794) -> (41.2033, 22.9733) centre (0, 0) ccw
  spline S170 degree 3 poles (41.7423, 18.5711) (41.6974, 18.5222) (41.6624, 18.465) (41.6164, 18.3404) (41.6058, 18.2742) (41.6106, 18.1414) (41.6259, 18.0762) (41.6807, 17.9552) (41.7196, 17.9006) (41.8162, 17.8095) (41.873, 17.7738) (41.9916, 17.7282) (42.0517, 17.7167) (42.1123, 17.7161) knots 0 0 0 0 0.019923 0.019923 0.039846 0.039846 0.059769 0.059769 0.079691 0.079691 0.099614 0.099614 0.117812 0.117812 0.117812 0.117812
  arc A121 (30.9045, 23.0839) -> (29.5622, 24.7297) centre (0.7975, -0.1016) ccw
  line L68 (29.6354, 8.1675) -> (37.3255, 10.3726)
  spline S171 degree 5 poles (41.2033, 22.9733) (41.1867, 22.9727) (41.1536, 22.9716) (41.104, 22.9699) (41.0379, 22.9674) (40.9554, 22.964) (40.873, 22.9602) (40.7907, 22.9561) (40.7084, 22.9517) (40.6263, 22.947) (40.5443, 22.942) (40.4624, 22.9366) (40.3805, 22.9309) (40.2988, 22.9249) (40.2172, 22.9185) (40.1357, 22.9118) (40.0544, 22.9048) (39.9731, 22.8975) (39.892, 22.8898) (39.8109, 22.8817) (39.73, 22.8733) (39.6636, 22.8662) (39.6135, 22.8606) (39.5795, 22.8567) (39.5616, 22.8546) (39.5598, 22.8544) knots -1 -1 -1 -1 -1 -1 -0.985714 -0.971429 -0.957143 -0.942857 -0.928571 -0.914286 -0.9 -0.885714 -0.871429 -0.857143 -0.842857 -0.828571 -0.814286 -0.8 -0.785714 -0.771429 -0.757143 -0.742857 -0.728571 -0.714286 -0.712736 -0.712736 -0.712736 -0.712736 -0.712736 -0.712736
  arc A122 (35.7247, 14.8682) -> (34.8338, 16.7961) centre (0.7975, -0.1016) ccw
  spline S172 degree 5 poles (43.7407, 13.1929) (43.7421, 13.1941) (43.7558, 13.2057) (43.7819, 13.2278) (43.8203, 13.2606) (43.871, 13.3041) (43.9325, 13.3573) (43.9938, 13.4109) (44.055, 13.4647) (44.116, 13.5189) (44.1768, 13.5735) (44.2375, 13.6283) (44.298, 13.6834) (44.3583, 13.7389) (44.4185, 13.7946) (44.4785, 13.8506) (44.5383, 13.907) (44.5979, 13.9636) (44.6574, 14.0206) (44.7168, 14.0778) (44.7759, 14.1353) (44.8349, 14.1931) (44.882, 14.2396) (44.9172, 14.2745) (44.9406, 14.2979) (44.9524, 14.3096) knots 0.712736 0.712736 0.712736 0.712736 0.712736 0.712736 0.714286 0.728571 0.742857 0.757143 0.771429 0.785714 0.8 0.814286 0.828571 0.842857 0.857143 0.871429 0.885714 0.9 0.914286 0.928571 0.942857 0.957143 0.971429 0.985714 1 1 1 1 1 1
  spline S173 degree 3 poles (40.4939, 21.1555) (40.4521, 21.1038) (40.4208, 21.0445) (40.3827, 20.9173) (40.3763, 20.8506) (40.3894, 20.7184) (40.4087, 20.6542) (40.471, 20.5369) (40.5133, 20.4849) (40.6155, 20.4) (40.6743, 20.3679) (40.7956, 20.3299) (40.8562, 20.3222) (40.9168, 20.3254) knots 0 0 0 0 0.019923 0.019923 0.039846 0.039846 0.059769 0.059769 0.079691 0.079691 0.099614 0.099614 0.117812 0.117812 0.117812 0.117812
  spline S174 degree 5 poles (43.7577, 17.628) (43.7412, 17.6295) (43.7082, 17.6326) (43.6588, 17.6371) (43.5929, 17.6429) (43.5106, 17.6498) (43.4284, 17.6564) (43.3462, 17.6627) (43.264, 17.6686) (43.182, 17.6743) (43.1, 17.6795) (43.018, 17.6845) (42.9361, 17.6891) (42.8543, 17.6933) (42.7726, 17.6973) (42.6909, 17.7008) (42.6093, 17.7041) (42.5277, 17.707) (42.4462, 17.7095) (42.3648, 17.7117) (42.2835, 17.7135) (42.2168, 17.7147) (42.1663, 17.7154) (42.1321, 17.7158) (42.1141, 17.716) (42.1123, 17.7161) knots -1 -1 -1 -1 -1 -1 -0.985714 -0.971429 -0.957143 -0.942857 -0.928571 -0.914286 -0.9 -0.885714 -0.871429 -0.857143 -0.842857 -0.828571 -0.814286 -0.8 -0.785714 -0.771429 -0.757143 -0.742857 -0.728571 -0.714286 -0.712736 -0.712736 -0.712736 -0.712736 -0.712736 -0.712736
  spline S175 degree 5 poles (-15.9134, 42.826) (-15.9146, 42.8273) (-15.9271, 42.8403) (-15.9508, 42.8649) (-15.9859, 42.9012) (-16.0325, 42.9491) (-16.0895, 43.0071) (-16.1468, 43.065) (-16.2044, 43.1226) (-16.2623, 43.1801) (-16.3206, 43.2374) (-16.3791, 43.2945) (-16.4379, 43.3514) (-16.497, 43.4081) (-16.5564, 43.4646) (-16.6161, 43.521) (-16.6761, 43.5772) (-16.7364, 43.6332) (-16.7969, 43.689) (-16.8578, 43.7446) (-16.9189, 43.8) (-16.9803, 43.8553) (-17.0296, 43.8993) (-17.0668, 43.9323) (-17.0916, 43.9542) (-17.104, 43.9652) knots 0.712736 0.712736 0.712736 0.712736 0.712736 0.712736 0.714286 0.728571 0.742857 0.757143 0.771429 0.785714 0.8 0.814286 0.828571 0.842857 0.857143 0.871429 0.885714 0.9 0.914286 0.928571 0.942857 0.957143 0.971429 0.985714 1 1 1 1 1 1
  arc A123 (-47.0634, 3.2433) -> (-47.0988, 2.6809) centre (0, 0) ccw
  spline S176 degree 5 poles (36.1687, 30.2871) (36.1525, 30.2834) (36.1202, 30.2762) (36.0718, 30.2652) (36.0074, 30.2503) (35.927, 30.2315) (35.8467, 30.2124) (35.7666, 30.1929) (35.6866, 30.1732) (35.6069, 30.1532) (35.5272, 30.1329) (35.4478, 30.1122) (35.3685, 30.0913) (35.2893, 30.0701) (35.2104, 30.0485) (35.1316, 30.0267) (35.053, 30.0046) (34.9745, 29.9821) (34.8962, 29.9593) (34.8182, 29.9362) (34.7402, 29.9128) (34.6764, 29.8934) (34.6281, 29.8785) (34.5955, 29.8683) (34.5783, 29.8629) (34.5766, 29.8624) knots -1 -1 -1 -1 -1 -1 -0.985714 -0.971429 -0.957143 -0.942857 -0.928571 -0.914286 -0.9 -0.885714 -0.871429 -0.857143 -0.842857 -0.828571 -0.814286 -0.8 -0.785714 -0.771429 -0.757143 -0.742857 -0.728571 -0.714286 -0.712736 -0.712736 -0.712736 -0.712736 -0.712736 -0.712736
  spline S177 degree 5 poles (-12.0047, 45.622) (-12.0083, 45.6059) (-12.0154, 45.5735) (-12.0261, 45.525) (-12.0401, 45.4604) (-12.0573, 45.3796) (-12.0742, 45.2989) (-12.0907, 45.2181) (-12.1069, 45.1374) (-12.1228, 45.0566) (-12.1383, 44.9759) (-12.1534, 44.8953) (-12.1683, 44.8146) (-12.1828, 44.734) (-12.1969, 44.6533) (-12.2107, 44.5727) (-12.2241, 44.4922) (-12.2372, 44.4116) (-12.2499, 44.3311) (-12.2623, 44.2506) (-12.2743, 44.1702) (-12.2838, 44.1041) (-12.2909, 44.0541) (-12.2956, 44.0202) (-12.2981, 44.0024) (-12.2983, 44.0007) knots -1 -1 -1 -1 -1 -1 -0.985714 -0.971429 -0.957143 -0.942857 -0.928571 -0.914286 -0.9 -0.885714 -0.871429 -0.857143 -0.842857 -0.828571 -0.814286 -0.8 -0.785714 -0.771429 -0.757143 -0.742857 -0.728571 -0.714286 -0.712736 -0.712736 -0.712736 -0.712736 -0.712736 -0.712736
  arc A124 (-42.5645, 20.3407) -> (-42.8044, 19.8308) centre (0, 0) ccw
  spline S178 degree 5 poles (-35.8125, -28.3685) (-35.8133, -28.3701) (-35.8218, -28.3859) (-35.8379, -28.4161) (-35.8616, -28.4607) (-35.8927, -28.5198) (-35.9303, -28.5919) (-35.9676, -28.6643) (-36.0046, -28.7369) (-36.0414, -28.8098) (-36.0778, -28.8829) (-36.1141, -28.9562) (-36.15, -29.0297) (-36.1857, -29.1034) (-36.2211, -29.1774) (-36.2563, -29.2516) (-36.2911, -29.326) (-36.3258, -29.4006) (-36.3601, -29.4755) (-36.3942, -29.5505) (-36.4281, -29.6258) (-36.4616, -29.7012) (-36.4883, -29.7618) (-36.5081, -29.8073) (-36.5213, -29.8376) (-36.5279, -29.8528) knots 0.712736 0.712736 0.712736 0.712736 0.712736 0.712736 0.714286 0.728571 0.742857 0.757143 0.771429 0.785714 0.8 0.814286 0.828571 0.842857 0.857143 0.871429 0.885714 0.9 0.914286 0.928571 0.942857 0.957143 0.971429 0.985714 1 1 1 1 1 1
  spline S179 degree 5 poles (-37.5231, -26.0639) (-37.524, -26.0654) (-37.5335, -26.0807) (-37.5514, -26.1098) (-37.5779, -26.1528) (-37.6126, -26.2098) (-37.6547, -26.2794) (-37.6964, -26.3493) (-37.738, -26.4195) (-37.7792, -26.4899) (-37.8202, -26.5605) (-37.861, -26.6314) (-37.9015, -26.7025) (-37.9417, -26.7739) (-37.9817, -26.8455) (-38.0214, -26.9173) (-38.0609, -26.9894) (-38.1002, -27.0617) (-38.1392, -27.1342) (-38.1779, -27.207) (-38.2164, -27.28) (-38.2546, -27.3532) (-38.285, -27.4119) (-38.3077, -27.4561) (-38.3228, -27.4856) (-38.3303, -27.5003) knots 0.712736 0.712736 0.712736 0.712736 0.712736 0.712736 0.714286 0.728571 0.742857 0.757143 0.771429 0.785714 0.8 0.814286 0.828571 0.842857 0.857143 0.871429 0.885714 0.9 0.914286 0.928571 0.942857 0.957143 0.971429 0.985714 1 1 1 1 1 1
  arc A125 (-45.622, 12.0047) -> (-45.7622, 11.4588) centre (0, 0) ccw
  spline S180 degree 5 poles (-7.6067, 45.0493) (-7.6077, 45.0508) (-7.6175, 45.0659) (-7.6362, 45.0946) (-7.6639, 45.1368) (-7.7007, 45.1925) (-7.7458, 45.2602) (-7.7912, 45.3278) (-7.837, 45.3952) (-7.8831, 45.4625) (-7.9296, 45.5297) (-7.9764, 45.5967) (-8.0235, 45.6637) (-8.0709, 45.7305) (-8.1187, 45.7971) (-8.1668, 45.8637) (-8.2152, 45.9301) (-8.2639, 45.9964) (-8.3129, 46.0625) (-8.3623, 46.1286) (-8.4119, 46.1945) (-8.4619, 46.2602) (-8.5021, 46.3128) (-8.5324, 46.3521) (-8.5526, 46.3783) (-8.5628, 46.3914) knots 0.712736 0.712736 0.712736 0.712736 0.712736 0.712736 0.714286 0.728571 0.742857 0.757143 0.771429 0.785714 0.8 0.814286 0.828571 0.842857 0.857143 0.871429 0.885714 0.9 0.914286 0.928571 0.942857 0.957143 0.971429 0.985714 1 1 1 1 1 1
  spline S181 degree 3 poles (-31.9746, -32.6333) (-31.9508, -32.5713) (-31.9393, -32.5053) (-31.9424, -32.3725) (-31.9569, -32.307) (-32.0102, -32.1854) (-32.0485, -32.1303) (-32.144, -32.038) (-32.2003, -32.0016) (-32.3237, -31.9524) (-32.3896, -31.9401) (-32.5166, -31.9414) (-32.5767, -31.9528) (-32.6333, -31.9746) knots 0 0 0 0 0.019923 0.019923 0.039846 0.039846 0.059769 0.059769 0.079691 0.079691 0.099614 0.099614 0.117812 0.117812 0.117812 0.117812
  spline S182 degree 5 poles (-18.5711, 41.7423) (-18.5724, 41.7435) (-18.5856, 41.7557) (-18.6109, 41.7788) (-18.6481, 41.8128) (-18.6976, 41.8576) (-18.7582, 41.912) (-18.819, 41.9661) (-18.8801, 42.02) (-18.9415, 42.0738) (-19.0032, 42.1273) (-19.0652, 42.1806) (-19.1275, 42.2337) (-19.1901, 42.2866) (-19.2529, 42.3393) (-19.3161, 42.3918) (-19.3794, 42.4441) (-19.4431, 42.4962) (-19.5071, 42.5481) (-19.5713, 42.5997) (-19.6357, 42.6512) (-19.7005, 42.7025) (-19.7525, 42.7434) (-19.7916, 42.7739) (-19.8177, 42.7943) (-19.8308, 42.8044) knots 0.712736 0.712736 0.712736 0.712736 0.712736 0.712736 0.714286 0.728571 0.742857 0.757143 0.771429 0.785714 0.8 0.814286 0.828571 0.842857 0.857143 0.871429 0.885714 0.9 0.914286 0.928571 0.942857 0.957143 0.971429 0.985714 1 1 1 1 1 1
  spline S183 degree 5 poles (-26.0639, 37.5231) (-26.0654, 37.524) (-26.0807, 37.5335) (-26.1098, 37.5514) (-26.1528, 37.5779) (-26.2098, 37.6126) (-26.2794, 37.6547) (-26.3493, 37.6964) (-26.4195, 37.738) (-26.4899, 37.7792) (-26.5605, 37.8202) (-26.6314, 37.861) (-26.7025, 37.9015) (-26.7739, 37.9417) (-26.8455, 37.9817) (-26.9173, 38.0214) (-26.9894, 38.0609) (-27.0617, 38.1002) (-27.1342, 38.1392) (-27.207, 38.1779) (-27.28, 38.2164) (-27.3532, 38.2546) (-27.4119, 38.285) (-27.4561, 38.3077) (-27.4856, 38.3228) (-27.5003, 38.3303) knots 0.712736 0.712736 0.712736 0.712736 0.712736 0.712736 0.714286 0.728571 0.742857 0.757143 0.771429 0.785714 0.8 0.814286 0.828571 0.842857 0.857143 0.871429 0.885714 0.9 0.914286 0.928571 0.942857 0.957143 0.971429 0.985714 1 1 1 1 1 1
  spline S184 degree 5 poles (-29.8624, -34.5766) (-29.8629, -34.5783) (-29.8683, -34.5955) (-29.8785, -34.6281) (-29.8934, -34.6764) (-29.9128, -34.7402) (-29.9362, -34.8182) (-29.9593, -34.8962) (-29.9821, -34.9745) (-30.0046, -35.053) (-30.0267, -35.1316) (-30.0485, -35.2104) (-30.0701, -35.2893) (-30.0913, -35.3685) (-30.1122, -35.4478) (-30.1329, -35.5272) (-30.1532, -35.6069) (-30.1732, -35.6866) (-30.1929, -35.7666) (-30.2124, -35.8467) (-30.2315, -35.927) (-30.2503, -36.0074) (-30.2652, -36.0718) (-30.2762, -36.1202) (-30.2834, -36.1525) (-30.2871, -36.1687) knots 0.712736 0.712736 0.712736 0.712736 0.712736 0.712736 0.714286 0.728571 0.742857 0.757143 0.771429 0.785714 0.8 0.814286 0.828571 0.842857 0.857143 0.871429 0.885714 0.9 0.914286 0.928571 0.942857 0.957143 0.971429 0.985714 1 1 1 1 1 1
  spline S185 degree 5 poles (37.5231, 26.0639) (37.524, 26.0654) (37.5335, 26.0807) (37.5514, 26.1098) (37.5779, 26.1528) (37.6126, 26.2098) (37.6547, 26.2794) (37.6964, 26.3493) (37.738, 26.4195) (37.7792, 26.4899) (37.8202, 26.5605) (37.861, 26.6314) (37.9015, 26.7025) (37.9417, 26.7739) (37.9817, 26.8455) (38.0214, 26.9173) (38.0609, 26.9894) (38.1002, 27.0617) (38.1392, 27.1342) (38.1779, 27.207) (38.2164, 27.28) (38.2546, 27.3532) (38.285, 27.4119) (38.3077, 27.4561) (38.3228, 27.4856) (38.3303, 27.5003) knots 0.712736 0.712736 0.712736 0.712736 0.712736 0.712736 0.714286 0.728571 0.742857 0.757143 0.771429 0.785714 0.8 0.814286 0.828571 0.842857 0.857143 0.871429 0.885714 0.9 0.914286 0.928571 0.942857 0.957143 0.971429 0.985714 1 1 1 1 1 1
  spline S186 degree 5 poles (-37.9991, -27.9562) (-37.9827, -27.9536) (-37.95, -27.9484) (-37.901, -27.9405) (-37.8358, -27.9297) (-37.7543, -27.916) (-37.673, -27.9019) (-37.5918, -27.8875) (-37.5108, -27.8729) (-37.4299, -27.8579) (-37.3492, -27.8426) (-37.2686, -27.827) (-37.1881, -27.8111) (-37.1078, -27.7949) (-37.0277, -27.7784) (-36.9476, -27.7615) (-36.8678, -27.7444) (-36.7881, -27.7269) (-36.7085, -27.7091) (-36.6292, -27.6909) (-36.5499, -27.6725) (-36.485, -27.657) (-36.4359, -27.6452) (-36.4027, -27.6371) (-36.3852, -27.6328) (-36.3835, -27.6324) knots -1 -1 -1 -1 -1 -1 -0.985714 -0.971429 -0.957143 -0.942857 -0.928571 -0.914286 -0.9 -0.885714 -0.871429 -0.857143 -0.842857 -0.828571 -0.814286 -0.8 -0.785714 -0.771429 -0.757143 -0.742857 -0.728571 -0.714286 -0.712736 -0.712736 -0.712736 -0.712736 -0.712736 -0.712736
  spline S187 degree 5 poles (-25.2933, -38.0467) (-25.2936, -38.0485) (-25.2968, -38.0662) (-25.3028, -38.0999) (-25.3115, -38.1496) (-25.3229, -38.2154) (-25.3363, -38.2956) (-25.3494, -38.376) (-25.3622, -38.4565) (-25.3747, -38.5371) (-25.3868, -38.6179) (-25.3986, -38.6988) (-25.41, -38.7798) (-25.4212, -38.861) (-25.432, -38.9423) (-25.4425, -39.0237) (-25.4527, -39.1053) (-25.4626, -39.1869) (-25.4721, -39.2687) (-25.4813, -39.3506) (-25.4903, -39.4327) (-25.4989, -39.5148) (-25.5055, -39.5806) (-25.5104, -39.63) (-25.5135, -39.663) (-25.5151, -39.6795) knots 0.712736 0.712736 0.712736 0.712736 0.712736 0.712736 0.714286 0.728571 0.742857 0.757143 0.771429 0.785714 0.8 0.814286 0.828571 0.842857 0.857143 0.871429 0.885714 0.9 0.914286 0.928571 0.942857 0.957143 0.971429 0.985714 1 1 1 1 1 1
  spline S188 degree 5 poles (-13.1929, 43.7407) (-13.1941, 43.7421) (-13.2057, 43.7558) (-13.2278, 43.7819) (-13.2606, 43.8203) (-13.3041, 43.871) (-13.3573, 43.9325) (-13.4109, 43.9938) (-13.4647, 44.055) (-13.5189, 44.116) (-13.5735, 44.1768) (-13.6283, 44.2375) (-13.6834, 44.298) (-13.7389, 44.3583) (-13.7946, 44.4185) (-13.8506, 44.4785) (-13.907, 44.5383) (-13.9636, 44.5979) (-14.0206, 44.6574) (-14.0778, 44.7168) (-14.1353, 44.7759) (-14.1931, 44.8349) (-14.2396, 44.882) (-14.2745, 44.9172) (-14.2979, 44.9406) (-14.3096, 44.9524) knots 0.712736 0.712736 0.712736 0.712736 0.712736 0.712736 0.714286 0.728571 0.742857 0.757143 0.771429 0.785714 0.8 0.814286 0.828571 0.842857 0.857143 0.871429 0.885714 0.9 0.914286 0.928571 0.942857 0.957143 0.971429 0.985714 1 1 1 1 1 1
  arc A126 (34.5814, 32.0875) -> (34.1956, 32.4983) centre (0, 0) ccw
  spline S189 degree 3 poles (-28.3685, 35.8125) (-28.31, 35.7811) (-28.2459, 35.7615) (-28.1138, 35.7479) (-28.047, 35.7541) (-27.9196, 35.7917) (-27.8602, 35.8228) (-27.7566, 35.9059) (-27.7135, 35.9572) (-27.6492, 36.0735) (-27.6288, 36.1373) (-27.6141, 36.2635) (-27.6179, 36.3246) (-27.6324, 36.3835) knots 0 0 0 0 0.019923 0.019923 0.039846 0.039846 0.059769 0.059769 0.079691 0.079691 0.099614 0.099614 0.117812 0.117812 0.117812 0.117812
  spline S190 degree 3 poles (25.2933, 38.0467) (25.2816, 37.9814) (25.2827, 37.9143) (25.3107, 37.7845) (25.3372, 37.7229) (25.4123, 37.6134) (25.4602, 37.5665) (25.5713, 37.4937) (25.6334, 37.4685) (25.7638, 37.4433) (25.8309, 37.4436) (25.9554, 37.4686) (26.0123, 37.4911) (26.0639, 37.5231) knots 0 0 0 0 0.019923 0.019923 0.039846 0.039846 0.059769 0.059769 0.079691 0.079691 0.099614 0.099614 0.117812 0.117812 0.117812 0.117812
  spline S191 degree 3 poles (-35.8125, -28.3685) (-35.7811, -28.31) (-35.7615, -28.2459) (-35.7479, -28.1138) (-35.7541, -28.047) (-35.7917, -27.9196) (-35.8228, -27.8602) (-35.9059, -27.7566) (-35.9572, -27.7135) (-36.0735, -27.6492) (-36.1373, -27.6288) (-36.2635, -27.6141) (-36.3246, -27.6179) (-36.3835, -27.6324) knots 0 0 0 0 0.019923 0.019923 0.039846 0.039846 0.059769 0.059769 0.079691 0.079691 0.099614 0.099614 0.117812 0.117812 0.117812 0.117812
  spline S192 degree 3 poles (-10.4204, 44.4828) (-10.3808, 44.4295) (-10.3311, 44.3845) (-10.2174, 44.3159) (-10.1543, 44.2931) (-10.0231, 44.2729) (-9.9561, 44.2757) (-9.827, 44.3069) (-9.7661, 44.3349) (-9.6584, 44.4127) (-9.6127, 44.4618) (-9.5457, 44.5698) (-9.5232, 44.6266) (-9.5112, 44.686) knots 0 0 0 0 0.019923 0.019923 0.039846 0.039846 0.059769 0.059769 0.079691 0.079691 0.099614 0.099614 0.117812 0.117812 0.117812 0.117812
  spline S193 degree 5 poles (-27.5003, -38.3303) (-27.4856, -38.3228) (-27.4561, -38.3077) (-27.4119, -38.285) (-27.3532, -38.2546) (-27.28, -38.2164) (-27.207, -38.1779) (-27.1342, -38.1392) (-27.0617, -38.1002) (-26.9894, -38.0609) (-26.9173, -38.0214) (-26.8455, -37.9817) (-26.7739, -37.9417) (-26.7025, -37.9015) (-26.6314, -37.861) (-26.5605, -37.8202) (-26.4899, -37.7792) (-26.4195, -37.738) (-26.3493, -37.6964) (-26.2794, -37.6547) (-26.2098, -37.6126) (-26.1528, -37.5779) (-26.1098, -37.5514) (-26.0807, -37.5335) (-26.0654, -37.524) (-26.0639, -37.5231) knots -1 -1 -1 -1 -1 -1 -0.985714 -0.971429 -0.957143 -0.942857 -0.928571 -0.914286 -0.9 -0.885714 -0.871429 -0.857143 -0.842857 -0.828571 -0.814286 -0.8 -0.785714 -0.771429 -0.757143 -0.742857 -0.728571 -0.714286 -0.712736 -0.712736 -0.712736 -0.712736 -0.712736 -0.712736
  spline S194 degree 5 poles (20.3254, 40.9168) (20.3254, 40.9186) (20.3264, 40.9365) (20.3281, 40.9707) (20.3305, 41.0211) (20.3335, 41.0878) (20.3368, 41.1691) (20.3398, 41.2505) (20.3423, 41.332) (20.3446, 41.4135) (20.3465, 41.4952) (20.3481, 41.5769) (20.3493, 41.6588) (20.3502, 41.7407) (20.3507, 41.8227) (20.3509, 41.9048) (20.3508, 41.987) (20.3504, 42.0693) (20.3496, 42.1516) (20.3485, 42.234) (20.347, 42.3165) (20.3453, 42.3991) (20.3436, 42.4652) (20.3422, 42.5148) (20.3413, 42.5479) (20.3407, 42.5645) knots 0.712736 0.712736 0.712736 0.712736 0.712736 0.712736 0.714286 0.728571 0.742857 0.757143 0.771429 0.785714 0.8 0.814286 0.828571 0.842857 0.857143 0.871429 0.885714 0.9 0.914286 0.928571 0.942857 0.957143 0.971429 0.985714 1 1 1 1 1 1
  arc A127 (-38.3303, -27.5003) -> (-37.9991, -27.9562) centre (0, 0) ccw
  line L69 (16.1588, 25.6672) -> (20.2551, 32.5389)
  spline S195 degree 5 poles (29.8528, 36.5279) (29.8376, 36.5213) (29.8073, 36.5081) (29.7618, 36.4883) (29.7012, 36.4616) (29.6258, 36.4281) (29.5505, 36.3942) (29.4755, 36.3601) (29.4006, 36.3258) (29.326, 36.2911) (29.2516, 36.2563) (29.1774, 36.2211) (29.1034, 36.1857) (29.0297, 36.15) (28.9562, 36.1141) (28.8829, 36.0778) (28.8098, 36.0414) (28.7369, 36.0046) (28.6643, 35.9676) (28.5919, 35.9303) (28.5198, 35.8927) (28.4607, 35.8616) (28.4161, 35.8379) (28.3859, 35.8218) (28.3701, 35.8133) (28.3685, 35.8125) knots -1 -1 -1 -1 -1 -1 -0.985714 -0.971429 -0.957143 -0.942857 -0.928571 -0.914286 -0.9 -0.885714 -0.871429 -0.857143 -0.842857 -0.828571 -0.814286 -0.8 -0.785714 -0.771429 -0.757143 -0.742857 -0.728571 -0.714286 -0.712736 -0.712736 -0.712736 -0.712736 -0.712736 -0.712736
  spline S196 degree 3 poles (-26.0639, 37.5231) (-26.0074, 37.4881) (-25.9447, 37.4645) (-25.8136, 37.4427) (-25.7466, 37.4446) (-25.6171, 37.4742) (-25.5559, 37.5014) (-25.4473, 37.5779) (-25.401, 37.6264) (-25.3296, 37.7384) (-25.3052, 37.8008) (-25.2826, 37.9259) (-25.2826, 37.987) (-25.2933, 38.0467) knots 0 0 0 0 0.019923 0.019923 0.039846 0.039846 0.059769 0.059769 0.079691 0.079691 0.099614 0.099614 0.117812 0.117812 0.117812 0.117812
  spline S197 degree 3 poles (31.9746, 32.6333) (31.9508, 32.5713) (31.9393, 32.5053) (31.9424, 32.3725) (31.9569, 32.307) (32.0102, 32.1854) (32.0485, 32.1303) (32.144, 32.038) (32.2003, 32.0016) (32.3237, 31.9524) (32.3896, 31.9401) (32.5166, 31.9414) (32.5767, 31.9528) (32.6333, 31.9746) knots 0 0 0 0 0.019923 0.019923 0.039846 0.039846 0.059769 0.059769 0.079691 0.079691 0.099614 0.099614 0.117812 0.117812 0.117812 0.117812
  arc A128 (-27.5003, 38.3303) -> (-27.9562, 37.9991) centre (0, 0) ccw
  arc A129 (-46.7669, 6.192) -> (-46.8375, 5.6329) centre (0, 0) ccw
  arc A130 (-20.4518, 31.4018) -> (-22.1786, 30.1655) centre (0.7975, -0.1016) ccw
  spline S198 degree 5 poles (-14.8456, 44.7782) (-14.8482, 44.7619) (-14.8533, 44.7291) (-14.8609, 44.6801) (-14.8709, 44.6147) (-14.8829, 44.533) (-14.8947, 44.4513) (-14.9061, 44.3697) (-14.9172, 44.2881) (-14.928, 44.2065) (-14.9384, 44.125) (-14.9485, 44.0436) (-14.9582, 43.9621) (-14.9676, 43.8807) (-14.9766, 43.7994) (-14.9853, 43.7181) (-14.9937, 43.6368) (-15.0017, 43.5556) (-15.0093, 43.4745) (-15.0166, 43.3934) (-15.0235, 43.3123) (-15.0289, 43.2458) (-15.0328, 43.1954) (-15.0354, 43.1613) (-15.0367, 43.1434) (-15.0368, 43.1416) knots -1 -1 -1 -1 -1 -1 -0.985714 -0.971429 -0.957143 -0.942857 -0.928571 -0.914286 -0.9 -0.885714 -0.871429 -0.857143 -0.842857 -0.828571 -0.814286 -0.8 -0.785714 -0.771429 -0.757143 -0.742857 -0.728571 -0.714286 -0.712736 -0.712736 -0.712736 -0.712736 -0.712736 -0.712736
  spline S199 degree 5 poles (39.6795, 25.5151) (39.663, 25.5135) (39.63, 25.5104) (39.5806, 25.5055) (39.5148, 25.4989) (39.4327, 25.4903) (39.3506, 25.4813) (39.2687, 25.4721) (39.1869, 25.4626) (39.1053, 25.4527) (39.0237, 25.4425) (38.9423, 25.432) (38.861, 25.4212) (38.7798, 25.41) (38.6988, 25.3986) (38.6179, 25.3868) (38.5371, 25.3747) (38.4565, 25.3622) (38.376, 25.3494) (38.2956, 25.3363) (38.2154, 25.3229) (38.1496, 25.3115) (38.0999, 25.3028) (38.0662, 25.2968) (38.0485, 25.2936) (38.0467, 25.2933) knots -1 -1 -1 -1 -1 -1 -0.985714 -0.971429 -0.957143 -0.942857 -0.928571 -0.914286 -0.9 -0.885714 -0.871429 -0.857143 -0.842857 -0.828571 -0.814286 -0.8 -0.785714 -0.771429 -0.757143 -0.742857 -0.728571 -0.714286 -0.712736 -0.712736 -0.712736 -0.712736 -0.712736 -0.712736
  spline S200 degree 5 poles (-45.7622, 11.4588) (-45.7497, 11.4479) (-45.7249, 11.426) (-45.6875, 11.3933) (-45.6376, 11.3499) (-45.5751, 11.2959) (-45.5125, 11.2422) (-45.4497, 11.1888) (-45.3867, 11.1357) (-45.3236, 11.083) (-45.2604, 11.0305) (-45.197, 10.9783) (-45.1334, 10.9265) (-45.0698, 10.8749) (-45.0059, 10.8237) (-44.9419, 10.7728) (-44.8778, 10.7222) (-44.8135, 10.6719) (-44.7491, 10.622) (-44.6845, 10.5724) (-44.6198, 10.5231) (-44.5665, 10.4829) (-44.5261, 10.4526) (-44.4987, 10.4322) (-44.4842, 10.4215) (-44.4828, 10.4204) knots -1 -1 -1 -1 -1 -1 -0.985714 -0.971429 -0.957143 -0.942857 -0.928571 -0.914286 -0.9 -0.885714 -0.871429 -0.857143 -0.842857 -0.828571 -0.814286 -0.8 -0.785714 -0.771429 -0.757143 -0.742857 -0.728571 -0.714286 -0.712736 -0.712736 -0.712736 -0.712736 -0.712736 -0.712736
  arc A131 (-39.9814, -25.0393) -> (-39.6795, -25.5151) centre (0, 0) ccw
  spline S201 degree 5 poles (35.8125, 28.3685) (35.8133, 28.3701) (35.8218, 28.3859) (35.8379, 28.4161) (35.8616, 28.4607) (35.8927, 28.5198) (35.9303, 28.5919) (35.9676, 28.6643) (36.0046, 28.7369) (36.0414, 28.8098) (36.0778, 28.8829) (36.1141, 28.9562) (36.15, 29.0297) (36.1857, 29.1034) (36.2211, 29.1774) (36.2563, 29.2516) (36.2911, 29.326) (36.3258, 29.4006) (36.3601, 29.4755) (36.3942, 29.5505) (36.4281, 29.6258) (36.4616, 29.7012) (36.4883, 29.7618) (36.5081, 29.8073) (36.5213, 29.8376) (36.5279, 29.8528) knots 0.712736 0.712736 0.712736 0.712736 0.712736 0.712736 0.714286 0.728571 0.742857 0.757143 0.771429 0.785714 0.8 0.814286 0.828571 0.842857 0.857143 0.871429 0.885714 0.9 0.914286 0.928571 0.942857 0.957143 0.971429 0.985714 1 1 1 1 1 1
  line L70 (-20.4896, -21.2406) -> (-26.1662, -26.8777)